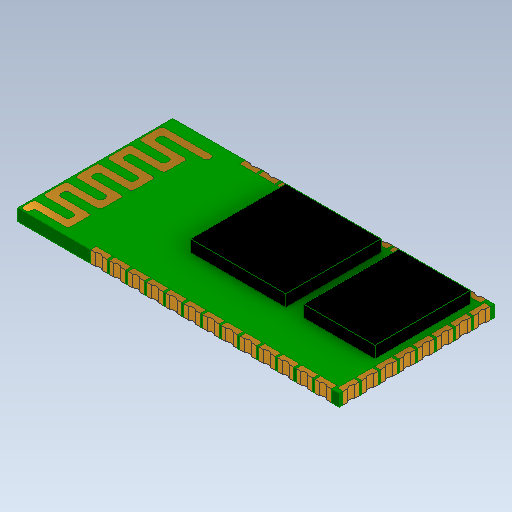
# Autodesk Inventor part: HC-05
Saved by Autodesk Inventor 2020 (Build 240168000, 168)
## iProperties
Created: 2019-12-28
Part Number: HC-05
Material: Generic
Document SubType Name: Modeling
Designer: ermoz
Density: 1 g/cm^3
Appearance: Default
Mass: 0.461242 g
Surface Area: 10.6929 cm^2
Volume: 0.461242 cm^3
Author: ermoz
Autodesk Inventor part; units mm, degrees
ref_plane "YZ Plane" through (0, 0, 0) normal (1, 0, 0) x (0, 1, 0)
ref_plane "XZ Plane" through (0, 0, 0) normal (0, 1, 0) x (-1, 0, 0)
ref_plane "XY Plane" through (0, 0, 0) normal (0, 0, 1) x (1, 0, 0)
sketch "Sketch1" plane through (0, 0, 0) normal (0, 1, 0) x (-1, 0, 0)
  line L0 (0, 0) -> (-27, 0)
  line L1 (-27, 0) -> (-27, -13)
  line L2 (-27, -13) -> (0, -13)
  line L3 (0, -13) -> (0, 0)
  dimension "d0" = 27
  dimension "d1" = 13
  constraints: 8 end point, 2 parallel, 1 horizontal, 1 perpendicular
  measures "d0" distance of L2.end L1.end
  measures "d1" distance of L1.end L0.end
extrude "Extrusion1" add sketch "Sketch1" along normal blind 1
sketch "Sketch2" plane through (0, 1, 0) normal (0, 1, 0) x (1, 0, 0)
  line L0 (27, 6.215) -> (26.5, 6.785) construction
  line L1 (26.5, 6.215) -> (27, 6.785) construction
  line L2 (26.5, 6.785) -> (26.5, 7.785)
  line L3 (26.5, 8.355) -> (26.5, 9.355)
  line L4 (26.5, 9.925) -> (26.5, 10.925)
  line L5 (26.5, 11.495) -> (26.5, 12.495)
  line L6 (27, 6.785) -> (27, 6.985)
  line L7 (27, 7.785) -> (27, 7.585)
  arc A0 (27, 7.585) -> (27, 6.985) centre (27.2975, 7.285) ccw
  line L8 (27, 8.355) -> (27, 8.555)
  line L9 (27, 9.355) -> (27, 9.155)
  arc A1 (27, 9.155) -> (27, 8.555) centre (27.2975, 8.855) ccw
  line L10 (27, 9.925) -> (27, 10.125)
  line L11 (27, 10.925) -> (27, 10.725)
  arc A2 (27, 10.725) -> (27, 10.125) centre (27.2975, 10.425) ccw
  line L12 (27, 11.495) -> (27, 11.695)
  line L13 (27, 12.495) -> (27, 12.295)
  arc A3 (27, 12.295) -> (27, 11.695) centre (27.2975, 11.995) ccw
  line L14 (26.5, 6.215) -> (26.5, 5.215)
  line L15 (26.5, 4.645) -> (26.5, 3.645)
  line L16 (26.5, 3.075) -> (26.5, 2.075)
  line L17 (26.5, 1.505) -> (26.5, 0.505)
  arc A4 (27, 6.015) -> (27, 5.415) centre (27.2975, 5.715) ccw
  arc A5 (27, 4.445) -> (27, 3.845) centre (27.2975, 4.145) ccw
  arc A6 (27, 2.875) -> (27, 2.275) centre (27.2975, 2.575) ccw
  arc A7 (27, 1.305) -> (27, 0.705) centre (27.2975, 1.005) ccw
  line L18 (27, 0.505) -> (27, 0.705)
  line L19 (27, 1.305) -> (27, 1.505)
  line L20 (27, 2.075) -> (27, 2.275)
  line L21 (27, 2.875) -> (27, 3.075)
  line L22 (27, 3.645) -> (27, 3.845)
  line L23 (27, 4.445) -> (27, 4.645)
  line L24 (27, 5.215) -> (27, 5.415)
  line L25 (27, 6.015) -> (27, 6.215)
  line L26 (27, 6.785) -> (27, 6.985)
  line L27 (27, 7.585) -> (27, 7.785)
  line L28 (27, 8.355) -> (27, 8.555)
  line L29 (27, 9.155) -> (27, 9.355)
  line L30 (27, 9.925) -> (27, 10.125)
  line L31 (27, 10.725) -> (27, 10.925)
  line L32 (27, 11.495) -> (27, 11.695)
  line L33 (27, 12.295) -> (27, 12.495)
  line L34 (27, 0.305) -> (26.5, 0.305)
  line L35 (26.5, 0.305) -> (26.5, 1.705)
  line L36 (26.5, 1.705) -> (27, 1.705)
  line L37 (27, 0.305) -> (26.5, 1.705) construction
  line L38 (26.5, 0.305) -> (27, 1.705) construction
  line L39 (27, 1.875) -> (26.5, 1.875)
  line L40 (26.5, 1.875) -> (26.5, 3.275)
  line L41 (26.5, 3.275) -> (27, 3.275)
  line L42 (27, 1.875) -> (26.5, 3.275) construction
  line L43 (26.5, 1.875) -> (27, 3.275) construction
  line L44 (27, 3.445) -> (26.5, 3.445)
  line L45 (26.5, 3.445) -> (26.5, 4.845)
  line L46 (26.5, 4.845) -> (27, 4.845)
  line L47 (27, 3.445) -> (26.5, 4.845) construction
  line L48 (26.5, 3.445) -> (27, 4.845) construction
  line L49 (27, 5.015) -> (26.5, 5.015)
  line L50 (26.5, 5.015) -> (26.5, 6.415)
  line L51 (26.5, 6.415) -> (27, 6.415)
  line L52 (27, 5.015) -> (26.5, 6.415) construction
  line L53 (26.5, 5.015) -> (27, 6.415) construction
  line L54 (27, 6.585) -> (26.5, 6.585)
  line L55 (26.5, 6.585) -> (26.5, 7.985)
  line L56 (26.5, 7.985) -> (27, 7.985)
  line L57 (27, 6.585) -> (26.5, 7.985) construction
  line L58 (26.5, 6.585) -> (27, 7.985) construction
  line L59 (27, 8.155) -> (26.5, 8.155)
  line L60 (26.5, 8.155) -> (26.5, 9.555)
  line L61 (26.5, 9.555) -> (27, 9.555)
  line L62 (27, 8.155) -> (26.5, 9.555) construction
  line L63 (26.5, 8.155) -> (27, 9.555) construction
  line L64 (27, 9.725) -> (26.5, 9.725)
  line L65 (26.5, 9.725) -> (26.5, 11.125)
  line L66 (26.5, 11.125) -> (27, 11.125)
  line L67 (27, 9.725) -> (26.5, 11.125) construction
  line L68 (26.5, 9.725) -> (27, 11.125) construction
  line L69 (27, 11.295) -> (26.5, 11.295)
  line L70 (26.5, 11.295) -> (26.5, 12.695)
  line L71 (26.5, 12.695) -> (27, 12.695)
  line L72 (27, 11.295) -> (26.5, 12.695) construction
  line L73 (26.5, 11.295) -> (27, 12.695) construction
  line L74 (27, 1.705) -> (27, 1.305)
  line L75 (27, 0.705) -> (27, 0.305)
  line L76 (27, 1.875) -> (27, 2.275)
  line L77 (27, 2.875) -> (27, 3.275)
  line L78 (27, 3.445) -> (27, 3.845)
  line L79 (27, 4.445) -> (27, 4.845)
  line L80 (27, 5.015) -> (27, 5.415)
  line L81 (27, 6.015) -> (27, 6.415)
  line L82 (27, 6.585) -> (27, 6.985)
  line L83 (27, 7.585) -> (27, 7.985)
  line L84 (27, 8.155) -> (27, 8.555)
  line L85 (27, 9.155) -> (27, 9.555)
  line L86 (27, 9.725) -> (27, 10.125)
  line L87 (27, 10.725) -> (27, 11.125)
  line L88 (27, 11.295) -> (27, 11.695)
  line L89 (27, 12.295) -> (27, 12.695)
  arc A8 (27, 1.305) -> (27, 0.705) centre (27.2975, 1.005) ccw
  arc A9 (27, 2.875) -> (27, 2.275) centre (27.2975, 2.575) ccw
  arc A10 (27, 4.445) -> (27, 3.845) centre (27.2975, 4.145) ccw
  arc A11 (27, 6.015) -> (27, 5.415) centre (27.2975, 5.715) ccw
  arc A12 (27, 7.585) -> (27, 6.985) centre (27.2975, 7.285) ccw
  arc A13 (27, 9.155) -> (27, 8.555) centre (27.2975, 8.855) ccw
  arc A14 (27, 10.725) -> (27, 10.125) centre (27.2975, 10.425) ccw
  line L90 (27, 0) -> (27, 13) projected
  arc A15 (27, 12.295) -> (27, 11.695) centre (27.2975, 11.995) ccw
  line L91 (27, 0.305) -> (27, 12.695)
  point P0 (0, 0)
  point P1 (26.75, 1.005)
  point P2 (26.75, 2.575)
  point P3 (26.75, 4.145)
  point P4 (26.75, 5.715)
  point P5 (26.75, 7.285)
  point P6 (26.75, 8.855)
  point P7 (26.75, 10.425)
  point P8 (26.75, 11.995)
  dimension "d6" = 0.57
  dimension "d8" = 1
  dimension "d12" = 1
  dimension "d16" = 1
  dimension "d19" = 0.5
  dimension "d20" = 1
  dimension "d22" = 0.2
  dimension "d23" = 0.2
  dimension "d24" = 0.2
  dimension "d25" = 0.2
  dimension "d29" = 1.4
  dimension "d30" = 1.4
  dimension "d31" = 1.4
  dimension "d32" = 1.4
  dimension "d33" = 1.4
  dimension "d34" = 1.4
  dimension "d35" = 1.4
  dimension "d36" = 1.4
  constraints: 182 end point, 32 point on circle, 16 centre point, 16 midpoint, 15 collinear, 8 coincident, 8 horizontal, 8 parallel, 8 perpendicular, 3 point on line, 1 vertical, 2 other
  measures "d6" distance of L1.start L0.end
  measures "d8" distance of L2.start L2.end
  measures "d12" distance of L3.start L3.end
  measures "d16" distance of L4.start L4.end
  measures "d19" distance of L5.end L13.start
  measures "d20" distance of L5.start L5.end
  measures "d22" distance of L7.start L7.end
  measures "d23" distance of L8.start L8.end
  measures "d24" distance of L9.start L9.end
  measures "d25" distance of L10.start L10.end
  measures "d29" distance of L34.end L35.end
  measures "d30" distance of L39.end L40.end
  measures "d31" distance of L44.end L45.end
  measures "d32" distance of L49.end L50.end
  measures "d33" distance of L54.end L55.end
  measures "d34" distance of L59.end L60.end
  measures "d35" distance of L64.end L65.end
  measures "d36" distance of L69.end L70.end
extrude "Extrusion2" cut sketch "Sketch2" against normal blind 1 contours L69 L70 L5 L71 L89 L13 A3 L12 L88 | L64 L65 L4 L66 L87 L11 A2 L10 L86 | L59 L60 L3 L61 L85 L9 A1 L8 L84 | L74 L19 A7 L18 L75 L34 L35 L17 L36 | L77 L21 A6 L20 L76 L39 L40 L16 L41 | L79 L23 A5 L22 L78 L44 L45 L15 L46 | L81 L25 A4 L24 L80 L49 L50 L14 L51 | L2 L55 L56 L83 L7 A0 L6 L82 L54
extrude "Extrusion3" add sketch "Sketch2" against normal blind 1 separate body contours L69 L70 L5 L71 L89 L13 A3 L12 L88 | L64 L65 L4 L66 L87 L11 A2 L10 L86 | L59 L60 L3 L61 L85 L9 A1 L8 L84 | L74 L19 A7 L18 L75 L34 L35 L17 L36 | L77 L21 A6 L20 L76 L39 L40 L16 L41 | L79 L23 A5 L22 L78 L44 L45 L15 L46 | L81 L25 A4 L24 L80 L49 L50 L14 L51 | L2 L55 L56 L83 L7 A0 L6 L82 L54
sketch "Sketch3" plane through (0, 1, 0) normal (0, 1, 0) x (1, 0, 0)
  line L0 (26.7293, 0.5191) -> (27.1446, 0.5191)
  line L1 (27.1446, 0.5191) -> (27.1446, 1.5386)
  line L2 (27.1446, 1.5386) -> (26.7293, 1.5386)
  line L3 (26.7293, 1.5386) -> (26.7293, 0.5191)
  line L4 (26.7293, 2.1711) -> (27.1446, 2.1711)
  line L5 (27.1446, 2.1711) -> (27.1446, 3.0584)
  line L6 (27.1446, 3.0584) -> (26.7293, 3.0584)
  line L7 (26.7293, 3.0584) -> (26.7293, 2.1711)
  line L8 (26.7293, 3.7192) -> (27.088, 3.7192)
  line L9 (27.088, 3.7192) -> (27.088, 4.616)
  line L10 (27.088, 4.616) -> (26.7293, 4.616)
  line L11 (26.7293, 4.616) -> (26.7293, 3.7192)
  line L12 (26.7293, 5.305) -> (27.1446, 5.305)
  line L13 (27.1446, 5.305) -> (27.1446, 6.1546)
  line L14 (27.1446, 6.1546) -> (26.7293, 6.1546)
  line L15 (26.7293, 6.1546) -> (26.7293, 5.305)
  line L16 (26.7293, 6.9192) -> (27.1446, 6.9192)
  line L17 (27.1446, 6.9192) -> (27.1446, 7.7122)
  line L18 (27.1446, 7.7122) -> (26.7293, 7.7122)
  line L19 (26.7293, 7.7122) -> (26.7293, 6.9192)
  line L20 (26.7293, 8.4673) -> (27.239, 8.4673)
  line L21 (27.239, 8.4673) -> (27.239, 9.3358)
  line L22 (27.239, 9.3358) -> (26.7293, 9.3358)
  line L23 (26.7293, 9.3358) -> (26.7293, 8.4673)
  line L24 (26.6726, 9.9966) -> (27.239, 9.9966)
  line L25 (27.239, 9.9966) -> (27.239, 10.8556)
  line L26 (27.239, 10.8556) -> (26.6726, 10.8556)
  line L27 (26.6726, 10.8556) -> (26.6726, 9.9966)
  line L28 (26.6726, 11.5541) -> (27.239, 11.5541)
  line L29 (27.239, 11.5541) -> (27.239, 12.517)
  line L30 (27.239, 12.517) -> (26.6726, 12.517)
  line L31 (26.6726, 12.517) -> (26.6726, 11.5541)
  point P0 (0, 0)
  constraints: 64 end point, 16 parallel, 11 point on line, 8 horizontal, 8 perpendicular
extrude "Extrusion4" cut sketch "Sketch3" against normal blind 1 bodies 1
sketch "Sketch4" plane through (0, 1, 0) normal (0, 1, 0) x (1, 0, 0)
  line L0 (24.93, 13) -> (24.93, 12.5)
  line L1 (24.93, 12.5) -> (26.33, 12.5)
  line L2 (26.33, 12.5) -> (26.33, 13)
  line L3 (23.36, 13) -> (23.36, 12.5)
  line L4 (23.36, 12.5) -> (24.76, 12.5)
  line L5 (24.76, 12.5) -> (24.76, 13)
  line L6 (21.79, 13) -> (21.79, 12.5)
  line L7 (21.79, 12.5) -> (23.19, 12.5)
  line L8 (23.19, 12.5) -> (23.19, 13)
  line L9 (20.22, 13) -> (20.22, 12.5)
  line L10 (20.22, 12.5) -> (21.62, 12.5)
  line L11 (21.62, 12.5) -> (21.62, 13)
  line L12 (18.65, 13) -> (18.65, 12.5)
  line L13 (18.65, 12.5) -> (20.05, 12.5)
  line L14 (20.05, 12.5) -> (20.05, 13)
  line L15 (17.08, 13) -> (17.08, 12.5)
  line L16 (17.08, 12.5) -> (18.48, 12.5)
  line L17 (18.48, 12.5) -> (18.48, 13)
  line L18 (15.51, 13) -> (15.51, 12.5)
  line L19 (15.51, 12.5) -> (16.91, 12.5)
  line L20 (16.91, 12.5) -> (16.91, 13)
  line L21 (13.94, 13) -> (13.94, 12.5)
  line L22 (13.94, 12.5) -> (15.34, 12.5)
  line L23 (15.34, 12.5) -> (15.34, 13)
  line L24 (12.37, 13) -> (12.37, 12.5)
  line L25 (12.37, 12.5) -> (13.77, 12.5)
  line L26 (13.77, 12.5) -> (13.77, 13)
  line L27 (10.8, 13) -> (10.8, 12.5)
  line L28 (10.8, 12.5) -> (12.2, 12.5)
  line L29 (12.2, 12.5) -> (12.2, 13)
  line L30 (9.23, 13) -> (9.23, 12.5)
  line L31 (9.23, 12.5) -> (10.63, 12.5)
  line L32 (10.63, 12.5) -> (10.63, 13)
  line L33 (7.66, 13) -> (7.66, 12.5)
  line L34 (7.66, 12.5) -> (9.06, 12.5)
  line L35 (9.06, 12.5) -> (9.06, 13)
  line L36 (6.09, 13) -> (6.09, 12.5)
  line L37 (6.09, 12.5) -> (7.49, 12.5)
  line L38 (7.49, 12.5) -> (7.49, 13)
  line L39 (26.33, 13) -> (25.93, 13)
  line L40 (24.93, 13) -> (25.33, 13)
  line L41 (24.76, 13) -> (24.36, 13)
  line L42 (23.36, 13) -> (23.76, 13)
  line L43 (23.19, 13) -> (22.79, 13)
  line L44 (21.79, 13) -> (22.19, 13)
  line L45 (21.62, 13) -> (21.22, 13)
  line L46 (20.22, 13) -> (20.62, 13)
  line L47 (20.05, 13) -> (19.65, 13)
  line L48 (18.65, 13) -> (19.05, 13)
  line L49 (18.48, 13) -> (18.08, 13)
  line L50 (17.08, 13) -> (17.48, 13)
  line L51 (16.91, 13) -> (16.51, 13)
  line L52 (15.51, 13) -> (15.91, 13)
  line L53 (15.34, 13) -> (14.94, 13)
  line L54 (13.94, 13) -> (14.34, 13)
  line L55 (13.77, 13) -> (13.37, 13)
  line L56 (12.37, 13) -> (12.77, 13)
  line L57 (12.2, 13) -> (11.8, 13)
  line L58 (10.8, 13) -> (11.2, 13)
  line L59 (10.63, 13) -> (10.23, 13)
  line L60 (9.23, 13) -> (9.63, 13)
  line L61 (9.06, 13) -> (8.66, 13)
  line L62 (7.66, 13) -> (8.06, 13)
  line L63 (7.49, 13) -> (7.09, 13)
  line L64 (6.09, 13) -> (6.49, 13)
  line L65 (6.09, 13) -> (6.09, 12.875)
  arc A0 (25.33, 13) -> (25.93, 13) centre (25.63, 13.2975) ccw
  arc A1 (23.76, 13) -> (24.36, 13) centre (24.06, 13.2975) ccw
  arc A2 (22.19, 13) -> (22.79, 13) centre (22.49, 13.2975) ccw
  arc A3 (20.62, 13) -> (21.22, 13) centre (20.92, 13.2975) ccw
  arc A4 (19.05, 13) -> (19.65, 13) centre (19.35, 13.2975) ccw
  arc A5 (17.48, 13) -> (18.08, 13) centre (17.78, 13.2975) ccw
  arc A6 (15.91, 13) -> (16.51, 13) centre (16.21, 13.2975) ccw
  arc A7 (14.34, 13) -> (14.94, 13) centre (14.64, 13.2975) ccw
  arc A8 (12.77, 13) -> (13.37, 13) centre (13.07, 13.2975) ccw
  arc A9 (11.2, 13) -> (11.8, 13) centre (11.5, 13.2975) ccw
  arc A10 (9.63, 13) -> (10.23, 13) centre (9.93, 13.2975) ccw
  arc A11 (8.06, 13) -> (8.66, 13) centre (8.36, 13.2975) ccw
  arc A12 (6.49, 13) -> (7.09, 13) centre (6.79, 13.2975) ccw
  line L66 (0, 13) -> (0, 0) projected
  line L67 (0, 6.5) -> (5.1876, 6.5)
  line L68 (24.93, 0) -> (24.93, 0.5)
  line L69 (24.93, 0.5) -> (26.33, 0.5)
  line L70 (26.33, 0.5) -> (26.33, 0)
  line L71 (23.36, 0) -> (23.36, 0.5)
  line L72 (23.36, 0.5) -> (24.76, 0.5)
  line L73 (24.76, 0.5) -> (24.76, 0)
  line L74 (21.79, 0) -> (21.79, 0.5)
  line L75 (21.79, 0.5) -> (23.19, 0.5)
  line L76 (23.19, 0.5) -> (23.19, 0)
  line L77 (20.22, 0) -> (20.22, 0.5)
  line L78 (20.22, 0.5) -> (21.62, 0.5)
  line L79 (21.62, 0.5) -> (21.62, 0)
  line L80 (18.65, 0) -> (18.65, 0.5)
  line L81 (18.65, 0.5) -> (20.05, 0.5)
  line L82 (20.05, 0.5) -> (20.05, 0)
  line L83 (17.08, 0) -> (17.08, 0.5)
  line L84 (17.08, 0.5) -> (18.48, 0.5)
  line L85 (18.48, 0.5) -> (18.48, 0)
  line L86 (15.51, 0) -> (15.51, 0.5)
  line L87 (15.51, 0.5) -> (16.91, 0.5)
  line L88 (16.91, 0.5) -> (16.91, 0)
  line L89 (13.94, 0) -> (13.94, 0.5)
  line L90 (13.94, 0.5) -> (15.34, 0.5)
  line L91 (15.34, 0.5) -> (15.34, 0)
  line L92 (12.37, 0) -> (12.37, 0.5)
  line L93 (12.37, 0.5) -> (13.77, 0.5)
  line L94 (13.77, 0.5) -> (13.77, 0)
  line L95 (10.8, 0.5) -> (12.2, 0.5)
  line L96 (12.2, 0.5) -> (12.2, 0)
  line L97 (9.23, 0) -> (9.23, 0.5)
  line L98 (9.23, 0.5) -> (10.63, 0.5)
  line L99 (10.63, 0.5) -> (10.63, 0)
  line L100 (7.66, 0) -> (7.66, 0.5)
  line L101 (7.66, 0.5) -> (9.06, 0.5)
  line L102 (9.06, 0.5) -> (9.06, 0)
  line L103 (6.09, 0) -> (6.09, 0.5)
  line L104 (6.09, 0.5) -> (7.49, 0.5)
  line L105 (7.49, 0.5) -> (7.49, 0)
  line L106 (26.33, 0) -> (25.93, 0)
  line L107 (24.93, 0) -> (25.33, 0)
  line L108 (24.76, 0) -> (24.36, 0)
  line L109 (23.36, 0) -> (23.76, 0)
  line L110 (23.19, 0) -> (22.79, 0)
  line L111 (21.79, 0) -> (22.19, 0)
  line L112 (21.62, 0) -> (21.22, 0)
  line L113 (20.22, 0) -> (20.62, 0)
  line L114 (20.05, 0) -> (19.65, 0)
  line L115 (18.65, 0) -> (19.05, 0)
  line L116 (18.48, 0) -> (18.08, 0)
  line L117 (17.08, 0) -> (17.48, 0)
  line L118 (16.91, 0) -> (16.51, 0)
  line L119 (15.51, 0) -> (15.91, 0)
  line L120 (15.34, 0) -> (14.94, 0)
  line L121 (13.94, 0) -> (14.34, 0)
  line L122 (13.77, 0) -> (13.37, 0)
  line L123 (12.37, 0) -> (12.77, 0)
  line L124 (12.2, 0) -> (11.8, 0)
  line L125 (10.8, 0) -> (11.2, 0)
  line L126 (10.63, 0) -> (10.23, 0)
  line L127 (9.23, 0) -> (9.63, 0)
  line L128 (9.06, 0) -> (8.66, 0)
  line L129 (7.66, 0) -> (8.06, 0)
  line L130 (7.49, 0) -> (7.09, 0)
  line L131 (6.09, 0) -> (6.49, 0)
  arc A13 (25.93, 0) -> (25.33, 0) centre (25.63, -0.2975) ccw
  arc A14 (24.36, 0) -> (23.76, 0) centre (24.06, -0.2975) ccw
  arc A15 (22.79, 0) -> (22.19, 0) centre (22.49, -0.2975) ccw
  arc A16 (21.22, 0) -> (20.62, 0) centre (20.92, -0.2975) ccw
  arc A17 (19.65, 0) -> (19.05, 0) centre (19.35, -0.2975) ccw
  arc A18 (18.08, 0) -> (17.48, 0) centre (17.78, -0.2975) ccw
  arc A19 (16.51, 0) -> (15.91, 0) centre (16.21, -0.2975) ccw
  arc A20 (14.94, 0) -> (14.34, 0) centre (14.64, -0.2975) ccw
  arc A21 (13.37, 0) -> (12.77, 0) centre (13.07, -0.2975) ccw
  arc A22 (11.8, 0) -> (11.2, 0) centre (11.5, -0.2975) ccw
  arc A23 (10.23, 0) -> (9.63, 0) centre (9.93, -0.2975) ccw
  arc A24 (8.66, 0) -> (8.06, 0) centre (8.36, -0.2975) ccw
  arc A25 (7.09, 0) -> (6.49, 0) centre (6.79, -0.2975) ccw
  line L132 (10.8, 0) -> (10.8, 0.5)
  line L133 (0, 0) -> (27, 0) projected
  dimension "d46" = 0.17
  dimension "d47" = 1.4
  dimension "d49" = 0.17
  dimension "d50" = 1.4
  dimension "d52" = 0.17
  dimension "d53" = 1.4
  dimension "d55" = 0.17
  dimension "d56" = 1.4
  dimension "d58" = 0.17
  dimension "d59" = 1.4
  dimension "d61" = 0.17
  dimension "d62" = 1.4
  dimension "d64" = 0.17
  dimension "d65" = 1.4
  dimension "d67" = 0.17
  dimension "d68" = 1.4
  dimension "d70" = 0.17
  dimension "d71" = 1.4
  dimension "d73" = 0.17
  dimension "d74" = 1.4
  dimension "d76" = 0.17
  dimension "d77" = 1.4
  dimension "d80" = 1.4
  dimension "d81" = 0.5
  dimension "d82" = 0.4
  dimension "d83" = 0.4
  dimension "d84" = 0.4
  dimension "d85" = 0.4
  dimension "d86" = 0.4
  dimension "d87" = 0.4
  dimension "d88" = 0.4
  dimension "d89" = 0.4
  dimension "d90" = 0.4
  dimension "d91" = 0.4
  dimension "d92" = 0.4
  dimension "d93" = 0.4
  dimension "d94" = 0.4
  dimension "d95" = 0.4
  dimension "d96" = 0.4
  dimension "d97" = 0.4
  dimension "d98" = 0.4
  dimension "d99" = 0.4
  dimension "d100" = 0.4
  dimension "d101" = 0.4
  dimension "d102" = 0.4
  dimension "d103" = 0.4
  dimension "d104" = 0.4
  dimension "d105" = 0.4
  dimension "d106" = 0.4
  dimension "d107" = 0.4
  dimension "d108" = 0.125
  constraints: 264 end point, 91 symmetric about line, 52 point on circle, 26 centre point, 13 parallel, 1 horizontal, 1 midpoint, 1 point on line, 1 vertical, 14 other
  measures "d46" distance of L0.start L5.end
  measures "d47" distance of L4.end L3.end
  measures "d49" distance of L3.start L8.end
  measures "d50" distance of L7.end L6.end
  measures "d52" distance of L6.start L11.end
  measures "d53" distance of L10.end L9.end
  measures "d55" distance of L9.start L14.end
  measures "d56" distance of L13.end L12.end
  measures "d58" distance of L12.start L17.end
  measures "d59" distance of L16.end L15.end
  measures "d61" distance of L15.start L20.end
  measures "d62" distance of L19.end L18.end
  measures "d64" distance of L18.start L23.end
  measures "d65" distance of L22.end L21.end
  measures "d67" distance of L21.start L26.end
  measures "d68" distance of L25.end L24.end
  measures "d70" distance of L24.start L29.end
  measures "d71" distance of L28.end L27.end
  measures "d73" distance of L27.start L32.end
  measures "d74" distance of L31.end L30.end
  measures "d76" distance of L30.start L35.end
  measures "d77" distance of L34.end L33.end
  measures "d80" distance of L37.end L36.end
  measures "d81" distance of L36.end L36.start
  measures "d82" distance of L2.end L39.end
  measures "d83" distance of L0.start L40.end
  measures "d84" distance of L5.end L41.end
  measures "d85" distance of L3.start L42.end
  measures "d86" distance of L8.end L43.end
  measures "d87" distance of L6.start L44.end
  measures "d88" distance of L11.end L45.end
  measures "d89" distance of L9.start L46.end
  measures "d90" distance of L14.end L47.end
  measures "d91" distance of L12.start L48.end
  measures "d92" distance of L17.end L49.end
  measures "d93" distance of L15.start L50.end
  measures "d94" distance of L20.end L51.end
  measures "d95" distance of L18.start L52.end
  measures "d96" distance of L23.end L53.end
  measures "d97" distance of L21.start L54.end
  measures "d98" distance of L26.end L55.end
  measures "d99" distance of L24.start L56.end
  measures "d100" distance of L29.end L57.end
  measures "d101" distance of L27.start L58.end
  measures "d102" distance of L32.end L59.end
  measures "d103" distance of L30.start L60.end
  measures "d104" distance of L35.end L61.end
  measures "d105" distance of L33.start L62.end
  measures "d106" distance of L38.end L63.end
  measures "d107" distance of L36.start L64.end
  measures "d108" distance of L36.start L65.end
extrude "Extrusion5" cut sketch "Sketch4" against normal blind 1 contours L40 A0 L39 L2 L1 L0 | L42 A1 L41 L5 L4 L3 | L44 A2 L43 L8 L7 L6 | L46 A3 L45 L11 L10 L9 | L48 A4 L47 L14 L13 L12 | L50 A5 L49 L17 L16 L15 | L52 A6 L51 L20 L19 L18 | L54 A7 L53 L23 L22 L21 | L56 A8 L55 L26 L25 L24 | L58 A9 L57 L29 L28 L27 | L60 A10 L59 L32 L31 L30 | L62 A11 L61 L35 L34 L33 | L64 A12 L63 L38 L37 L36 | L68 L69 L70 L106 A13 L107 | L130 A25 L131 L103 L104 L105 | L128 A24 L129 L100 L101 L102 | L126 A23 L127 L97 L98 L99 | L124 A22 L125 L132 L95 L96 | L122 A21 L123 L92 L93 L94 | L120 A20 L121 L89 L90 L91 | L118 A19 L119 L86 L87 L88 | L116 A18 L117 L83 L84 L85 | L114 A17 L115 L80 L81 L82 | L112 A16 L113 L77 L78 L79 | L110 A15 L111 L74 L75 L76 | L108 A14 L109 L71 L72 L73 bodies 1
extrude "Extrusion6" add sketch "Sketch4" against normal blind 1 separate body contours L40 A0 L39 L2 L1 L0 | L42 A1 L41 L5 L4 L3 | L44 A2 L43 L8 L7 L6 | L46 A3 L45 L11 L10 L9 | L48 A4 L47 L14 L13 L12 | L50 A5 L49 L17 L16 L15 | L52 A6 L51 L20 L19 L18 | L54 A7 L53 L23 L22 L21 | L56 A8 L55 L26 L25 L24 | L58 A9 L57 L29 L28 L27 | L60 A10 L59 L32 L31 L30 | L62 A11 L61 L35 L34 L33 | L64 A12 L63 L38 L37 L36 | L68 L69 L70 L106 A13 L107 | L130 A25 L131 L103 L104 L105 | L128 A24 L129 L100 L101 L102 | L126 A23 L127 L97 L98 L99 | L124 A22 L125 L132 L95 L96 | L122 A21 L123 L92 L93 L94 | L120 A20 L121 L89 L90 L91 | L118 A19 L119 L86 L87 L88 | L116 A18 L117 L83 L84 L85 | L114 A17 L115 L80 L81 L82 | L112 A16 L113 L77 L78 L79 | L110 A15 L111 L74 L75 L76 | L108 A14 L109 L71 L72 L73
sketch "Sketch5" plane through (0, 1, 0) normal (0, 1, 0) x (1, 0, 0)
  line L0 (6.3703, 13.1269) -> (7.3266, 13.1269)
  line L1 (7.3266, 13.1269) -> (7.3266, 12.766)
  line L2 (7.3266, 12.766) -> (6.3703, 12.766)
  line L3 (6.3703, 12.766) -> (6.3703, 13.1269)
  line L4 (7.904, 13.1269) -> (8.9866, 13.1269)
  line L5 (8.9866, 13.1269) -> (8.9866, 12.766)
  line L6 (8.9866, 12.766) -> (7.904, 12.766)
  line L7 (7.904, 12.766) -> (7.904, 13.1269)
  line L8 (9.4918, 13.2352) -> (10.5564, 13.2352)
  line L9 (10.5564, 13.2352) -> (10.5564, 12.766)
  line L10 (10.5564, 12.766) -> (9.4918, 12.766)
  line L11 (9.4918, 12.766) -> (9.4918, 13.2352)
  line L12 (11.0616, 13.2352) -> (11.9638, 13.2352)
  line L13 (11.9638, 13.2352) -> (11.9638, 12.766)
  line L14 (11.9638, 12.766) -> (11.0616, 12.766)
  line L15 (11.0616, 12.766) -> (11.0616, 13.2352)
  line L16 (12.5592, 13.2352) -> (13.6419, 13.2352)
  line L17 (13.6419, 13.2352) -> (13.6419, 12.6217)
  line L18 (13.6419, 12.6217) -> (12.5592, 12.6217)
  line L19 (12.5592, 12.6217) -> (12.5592, 13.2352)
  line L20 (14.2553, 13.2352) -> (15.1214, 13.2352)
  line L21 (15.1214, 13.2352) -> (15.1214, 12.766)
  line L22 (15.1214, 12.766) -> (14.2553, 12.766)
  line L23 (14.2553, 12.766) -> (14.2553, 13.2352)
  line L24 (15.7891, 13.2352) -> (16.6732, 13.2352)
  line L25 (16.6732, 13.2352) -> (16.6732, 12.766)
  line L26 (16.6732, 12.766) -> (15.7891, 12.766)
  line L27 (15.7891, 12.766) -> (15.7891, 13.2352)
  line L28 (17.3769, 13.2352) -> (18.225, 13.2352)
  line L29 (18.225, 13.2352) -> (18.225, 12.766)
  line L30 (18.225, 12.766) -> (17.3769, 12.766)
  line L31 (17.3769, 12.766) -> (17.3769, 13.2352)
  line L32 (18.8204, 13.2352) -> (19.903, 13.2352)
  line L33 (19.903, 13.2352) -> (19.903, 12.766)
  line L34 (19.903, 12.766) -> (18.8204, 12.766)
  line L35 (18.8204, 12.766) -> (18.8204, 13.2352)
  line L36 (20.4263, 13.2352) -> (21.5269, 13.2352)
  line L37 (21.5269, 13.2352) -> (21.5269, 12.766)
  line L38 (21.5269, 12.766) -> (20.4263, 12.766)
  line L39 (20.4263, 12.766) -> (20.4263, 13.2352)
  line L40 (22.0322, 13.2352) -> (23.0065, 13.2352)
  line L41 (23.0065, 13.2352) -> (23.0065, 12.766)
  line L42 (23.0065, 12.766) -> (22.0322, 12.766)
  line L43 (22.0322, 12.766) -> (22.0322, 13.2352)
  line L44 (23.6381, 13.2352) -> (24.5222, 13.2352)
  line L45 (24.5222, 13.2352) -> (24.5222, 12.766)
  line L46 (24.5222, 12.766) -> (23.6381, 12.766)
  line L47 (23.6381, 12.766) -> (23.6381, 13.2352)
  line L48 (25.13, 13.2352) -> (26.1281, 13.2352)
  line L49 (26.1281, 13.2352) -> (26.1281, 12.766)
  line L50 (26.1281, 12.766) -> (25.13, 12.766)
  line L51 (25.13, 12.766) -> (25.13, 13.2352)
  line L52 (6.2439, -0.2615) -> (7.3266, -0.2615)
  line L53 (7.3266, -0.2615) -> (7.3266, 0.2618)
  line L54 (7.3266, 0.2618) -> (6.2439, 0.2618)
  line L55 (6.2439, 0.2618) -> (6.2439, -0.2615)
  line L56 (7.904, 0.2618) -> (8.8964, 0.2618)
  line L57 (8.8964, 0.2618) -> (8.8964, -0.3878)
  line L58 (8.8964, -0.3878) -> (7.904, -0.3878)
  line L59 (7.904, -0.3878) -> (7.904, 0.2618)
  line L60 (9.4918, 0.2618) -> (10.4301, 0.2618)
  line L61 (10.4301, 0.2618) -> (10.4301, -0.3878)
  line L62 (10.4301, -0.3878) -> (9.4918, -0.3878)
  line L63 (9.4918, -0.3878) -> (9.4918, 0.2618)
  line L64 (11.0616, 0.2618) -> (12.0901, 0.2618)
  line L65 (12.0901, 0.2618) -> (12.0901, -0.2615)
  line L66 (12.0901, -0.2615) -> (11.0616, -0.2615)
  line L67 (11.0616, -0.2615) -> (11.0616, 0.2618)
  line L68 (12.5592, 0.2618) -> (13.6419, 0.2618)
  line L69 (13.6419, 0.2618) -> (13.6419, -0.2615)
  line L70 (13.6419, -0.2615) -> (12.5592, -0.2615)
  line L71 (12.5592, -0.2615) -> (12.5592, 0.2618)
  line L72 (14.2553, 0.2618) -> (15.1214, 0.2618)
  line L73 (15.1214, 0.2618) -> (15.1214, -0.2615)
  line L74 (15.1214, -0.2615) -> (14.2553, -0.2615)
  line L75 (14.2553, -0.2615) -> (14.2553, 0.2618)
  line L76 (15.7891, 0.2618) -> (16.6732, 0.2618)
  line L77 (16.6732, 0.2618) -> (16.6732, -0.3878)
  line L78 (16.6732, -0.3878) -> (15.7891, -0.3878)
  line L79 (15.7891, -0.3878) -> (15.7891, 0.2618)
  line L80 (17.3769, 0.2618) -> (18.3332, 0.2618)
  line L81 (18.3332, 0.2618) -> (18.3332, -0.3878)
  line L82 (18.3332, -0.3878) -> (17.3769, -0.3878)
  line L83 (17.3769, -0.3878) -> (17.3769, 0.2618)
  line L84 (18.8204, 0.2618) -> (19.903, 0.2618)
  line L85 (19.903, 0.2618) -> (19.903, -0.3878)
  line L86 (19.903, -0.3878) -> (18.8204, -0.3878)
  line L87 (18.8204, -0.3878) -> (18.8204, 0.2618)
  line L88 (20.5165, 0.2618) -> (21.5269, 0.2618)
  line L89 (21.5269, 0.2618) -> (21.5269, -0.3878)
  line L90 (21.5269, -0.3878) -> (20.5165, -0.3878)
  line L91 (20.5165, -0.3878) -> (20.5165, 0.2618)
  line L92 (22.0322, 0.2618) -> (23.0967, 0.2618)
  line L93 (23.0967, 0.2618) -> (23.0967, -0.3878)
  line L94 (23.0967, -0.3878) -> (22.0322, -0.3878)
  line L95 (22.0322, -0.3878) -> (22.0322, 0.2618)
  line L96 (23.6381, 0.2618) -> (24.6124, 0.2618)
  line L97 (24.6124, 0.2618) -> (24.6124, -0.3878)
  line L98 (24.6124, -0.3878) -> (23.6381, -0.3878)
  line L99 (23.6381, -0.3878) -> (23.6381, 0.2618)
  line L100 (25.13, 0.2618) -> (26.1281, 0.2618)
  line L101 (26.1281, 0.2618) -> (26.1281, -0.3878)
  line L102 (26.1281, -0.3878) -> (25.13, -0.3878)
  line L103 (25.13, -0.3878) -> (25.13, 0.2618)
  point P0 (0, 0)
  constraints: 208 end point, 63 point on line, 52 parallel, 26 horizontal, 26 perpendicular
extrude "Extrusion7" cut sketch "Sketch5" against normal blind 1 bodies 1
sketch "Sketch6" plane through (0, 1, 0) normal (0, 1, 0) x (1, 0, 0)
  line L0 (27, 13) -> (26, 13)
  line L1 (26, 13) -> (26, 12)
  line L2 (26, 12) -> (27, 12)
  line L3 (27, 12) -> (27, 13)
  line L4 (26, 12) -> (20, 12)
  line L5 (20, 12) -> (20, 4)
  line L6 (20, 4) -> (26, 4)
  line L7 (26, 4) -> (26, 12)
  line L8 (18.5, 12) -> (10.5, 12)
  line L9 (10.5, 12) -> (10.5, 4)
  line L10 (10.5, 4) -> (18.5, 4)
  line L11 (18.5, 4) -> (18.5, 12)
  point P0 (0, 0)
  dimension "d115" = 1
  dimension "d116" = 1
  dimension "d117" = 6
  dimension "d119" = 1.5
  dimension "d120" = 8
  dimension "d121" = 8
  constraints: 24 end point, 6 parallel, 3 horizontal, 3 perpendicular
  measures "d115" distance of L2.end L1.end
  measures "d116" distance of L1.end L0.end
  measures "d117" distance of L6.end L5.end
  measures "d119" distance of L4.end L8.start
  measures "d120" distance of L10.end L9.end
  measures "d121" distance of L9.end L8.end
extrude "Extrusion8" add sketch "Sketch6" along normal blind 1 contours L7 L6 L5 L4 | L11 L10 L9 L8 bodies 1
sketch "Sketch7" plane through (0, 1, 0) normal (0, 1, 0) x (1, 0, 0)
  line L0 (0.1, 12) -> (0.85, 12)
  line L1 (0.1, 11.25) -> (0.1, 12)
  line L2 (4.25, 12) -> (0.1, 12)
  line L3 (0.1, 11.75) -> (0.1, 11.34)
  line L4 (1.01, 11.34) -> (4.25, 11.34)
  line L5 (4.5, 11.59) -> (4.5, 11.75)
  line L6 (0.35, 12) -> (0.76, 12)
  line L7 (0.76, 11.09) -> (0.76, 10.91)
  line L8 (0.76, 10) -> (0.35, 10)
  line L9 (0.1, 10) -> (0.1, 12)
  line L10 (0.1, 10) -> (2.69, 10)
  line L11 (3.6, 10) -> (3.6, 10.66)
  line L12 (3.6, 10.66) -> (1.01, 10.66)
  line L13 (0.1, 10.66) -> (0.1, 10.25)
  line L14 (3.35, 10.66) -> (2.94, 10.66)
  line L15 (2.94, 9.75) -> (2.94, 9.57)
  line L16 (2.94, 8.66) -> (3.6, 8.66)
  line L17 (3.6, 8.66) -> (3.6, 10.41)
  line L18 (3.35, 8.66) -> (1.01, 8.66)
  line L19 (0.1, 8.66) -> (0.1, 9.07)
  line L20 (0.35, 9.32) -> (2.69, 9.32)
  line L21 (3.6, 9.32) -> (3.6, 8.91)
  line L22 (0.1, 9.32) -> (0.76, 9.32)
  line L23 (0.76, 8.41) -> (0.76, 8.23)
  line L24 (0.76, 7.32) -> (0.35, 7.32)
  line L25 (0.1, 7.57) -> (0.1, 9.32)
  line L26 (0.1, 7.32) -> (2.69, 7.32)
  line L27 (3.6, 7.32) -> (3.6, 7.73)
  line L28 (3.35, 7.98) -> (1.01, 7.98)
  line L29 (0.1, 7.98) -> (0.1, 7.32)
  line L30 (3.6, 7.98) -> (2.94, 7.98)
  line L31 (2.94, 7.07) -> (2.94, 6.89)
  line L32 (2.94, 5.98) -> (3.35, 5.98)
  line L33 (3.6, 6.23) -> (3.6, 7.98)
  line L34 (3.6, 5.98) -> (1.01, 5.98)
  line L35 (0.1, 5.98) -> (0.1, 6.39)
  line L36 (0.35, 6.64) -> (2.69, 6.64)
  line L37 (3.6, 6.64) -> (3.6, 5.98)
  line L38 (0.35, 6.64) -> (0.76, 6.64)
  line L39 (0.76, 5.73) -> (0.76, 5.55)
  line L40 (0.76, 4.64) -> (0.1, 4.64)
  line L41 (0.1, 4.89) -> (0.1, 6.64)
  line L42 (0.35, 4.64) -> (2.69, 4.64)
  line L43 (3.6, 4.64) -> (3.6, 5.05)
  line L44 (3.35, 5.3) -> (1.01, 5.3)
  line L45 (0.1, 5.3) -> (0.1, 4.64)
  line L46 (3.6, 5.3) -> (2.94, 5.3)
  line L47 (2.94, 4.39) -> (2.94, 4.21)
  line L48 (2.94, 3.3) -> (3.5, 3.3)
  line L49 (3.6, 3.55) -> (3.6, 5.3)
  line L50 (3.35, 3.3) -> (1.01, 3.3)
  line L51 (0.1, 3.3) -> (0.1, 3.71)
  line L52 (0.35, 3.96) -> (2.69, 3.96)
  line L53 (3.6, 3.96) -> (3.6, 3.3)
  line L54 (0.2, 3.96) -> (0.76, 3.96)
  line L55 (0.76, 3.05) -> (0.76, 2.87)
  line L56 (0.76, 1.96) -> (0.35, 1.96)
  line L57 (0.1, 2.21) -> (0.1, 3.96)
  line L58 (0.2, 1.96) -> (2.69, 1.96)
  line L59 (3.6, 1.96) -> (3.6, 2.37)
  line L60 (3.5, 2.62) -> (1.01, 2.62)
  line L61 (0.1, 2.62) -> (0.1, 2.06)
  line L62 (3.35, 2.62) -> (2.94, 2.62)
  line L63 (2.94, 1.71) -> (2.94, 1.53)
  line L64 (2.94, 0.62) -> (3.6, 0.62)
  line L65 (3.6, 0.87) -> (3.6, 2.62)
  line L66 (3.35, 0.62) -> (1.01, 0.62)
  line L67 (0.1, 0.62) -> (0.1, 1.03)
  line L68 (0.35, 1.28) -> (2.69, 1.28)
  line L69 (3.6, 1.28) -> (3.6, 0.72)
  line L70 (0.1, 0.62) -> (0.76, 0.62)
  line L71 (0.76, 0.37) -> (0.76, 0.35)
  line L72 (0.51, 0.1) -> (0.35, 0.1)
  line L73 (0.1, 0.35) -> (0.1, 0.62)
  arc A0 (0.1, 0.2) -> (0.2, 0.1) centre (0.2, 0.2) ccw
  arc A1 (0.66, 0.1) -> (0.76, 0.2) centre (0.66, 0.2) ccw
  arc A2 (0.2, 1.28) -> (0.1, 1.18) centre (0.2, 1.18) ccw
  arc A3 (0.86, 0.62) -> (0.76, 0.52) centre (0.86, 0.52) ccw
  arc A4 (3.5, 0.62) -> (3.6, 0.72) centre (3.5, 0.72) ccw
  arc A5 (2.84, 1.28) -> (2.94, 1.38) centre (2.84, 1.38) ccw
  arc A6 (3.6, 2.52) -> (3.5, 2.62) centre (3.5, 2.52) ccw
  arc A7 (2.94, 1.86) -> (2.84, 1.96) centre (2.84, 1.86) ccw
  arc A8 (0.1, 2.06) -> (0.2, 1.96) centre (0.2, 2.06) ccw
  arc A9 (0.76, 2.72) -> (0.86, 2.62) centre (0.86, 2.72) ccw
  arc A10 (0.86, 3.3) -> (0.76, 3.2) centre (0.86, 3.2) ccw
  arc A11 (0.2, 3.96) -> (0.1, 3.86) centre (0.2, 3.86) ccw
  arc A12 (2.84, 3.96) -> (2.94, 4.06) centre (2.84, 4.06) ccw
  arc A13 (3.5, 3.3) -> (3.6, 3.4) centre (3.5, 3.4) ccw
  arc A14 (0.35, 1.28) -> (0.1, 1.03) centre (0.35, 1.03) ccw
  arc A15 (0.1, 0.35) -> (0.35, 0.1) centre (0.35, 0.35) ccw
  arc A16 (0.51, 0.1) -> (0.76, 0.35) centre (0.51, 0.35) ccw
  arc A17 (2.69, 1.28) -> (2.94, 1.53) centre (2.69, 1.53) ccw
  arc A18 (3.35, 0.62) -> (3.6, 0.87) centre (3.35, 0.87) ccw
  arc A19 (1.01, 0.62) -> (0.76, 0.37) centre (1.01, 0.37) ccw
  arc A20 (2.94, 1.71) -> (2.69, 1.96) centre (2.69, 1.71) ccw
  arc A21 (3.6, 2.37) -> (3.35, 2.62) centre (3.35, 2.37) ccw
  arc A22 (0.76, 2.87) -> (1.01, 2.62) centre (1.01, 2.87) ccw
  arc A23 (1.01, 3.3) -> (0.76, 3.05) centre (1.01, 3.05) ccw
  arc A24 (0.1, 2.21) -> (0.35, 1.96) centre (0.35, 2.21) ccw
  arc A25 (0.35, 3.96) -> (0.1, 3.71) centre (0.35, 3.71) ccw
  arc A26 (3.35, 3.3) -> (3.6, 3.55) centre (3.35, 3.55) ccw
  arc A27 (2.69, 3.96) -> (2.94, 4.21) centre (2.69, 4.21) ccw
  arc A28 (2.94, 4.39) -> (2.69, 4.64) centre (2.69, 4.39) ccw
  arc A29 (3.6, 5.05) -> (3.35, 5.3) centre (3.35, 5.05) ccw
  arc A30 (0.76, 5.55) -> (1.01, 5.3) centre (1.01, 5.55) ccw
  arc A31 (0.1, 4.89) -> (0.35, 4.64) centre (0.35, 4.89) ccw
  arc A32 (0.35, 6.64) -> (0.1, 6.39) centre (0.35, 6.39) ccw
  arc A33 (1.01, 5.98) -> (0.76, 5.73) centre (1.01, 5.73) ccw
  arc A34 (0.35, 6.64) -> (0.1, 6.39) centre (0.35, 6.39) ccw
  arc A35 (2.69, 6.64) -> (2.94, 6.89) centre (2.69, 6.89) ccw
  arc A36 (3.35, 5.98) -> (3.6, 6.23) centre (3.35, 6.23) ccw
  arc A37 (2.94, 7.07) -> (2.69, 7.32) centre (2.69, 7.07) ccw
  arc A38 (3.6, 7.73) -> (3.35, 7.98) centre (3.35, 7.73) ccw
  arc A39 (3.35, 8.66) -> (3.6, 8.91) centre (3.35, 8.91) ccw
  arc A40 (2.69, 9.32) -> (2.94, 9.57) centre (2.69, 9.57) ccw
  arc A41 (1.01, 8.66) -> (0.76, 8.41) centre (1.01, 8.41) ccw
  arc A42 (0.35, 9.32) -> (0.1, 9.07) centre (0.35, 9.07) ccw
  arc A43 (0.1, 7.57) -> (0.35, 7.32) centre (0.35, 7.57) ccw
  arc A44 (0.76, 8.23) -> (1.01, 7.98) centre (1.01, 8.23) ccw
  arc A45 (3.6, 10.41) -> (3.35, 10.66) centre (3.35, 10.41) ccw
  arc A46 (2.94, 9.75) -> (2.69, 10) centre (2.69, 9.75) ccw
  arc A47 (0.76, 10.91) -> (1.01, 10.66) centre (1.01, 10.91) ccw
  arc A48 (0.1, 10.25) -> (0.35, 10) centre (0.35, 10.25) ccw
  arc A49 (0.35, 12) -> (0.1, 11.75) centre (0.35, 11.75) ccw
  arc A50 (1.01, 11.34) -> (0.76, 11.09) centre (1.01, 11.09) ccw
  arc A51 (4.25, 11.34) -> (4.5, 11.59) centre (4.25, 11.59) ccw
  arc A52 (4.5, 11.75) -> (4.25, 12) centre (4.25, 11.75) ccw
  arc A53 (0.35, 1.28) -> (0.1, 1.03) centre (0.35, 1.03) ccw
  point P0 (0, 13)
  point P1 (0.1, 1.96)
  dimension "d163" = 0.1
  dimension "d164" = 0.25
  dimension "d165" = 0.25
  constraints: 148 end point, 108 point on circle, 108 tangent, 99 point on line, 54 centre point, 51 equal radius, 36 parallel, 19 horizontal, 18 perpendicular
  measures "d163" radius of A0
  measures "d164" radius of A14
  measures "d165" radius of A37
extrude "Extrusion9" cut sketch "Sketch7" against normal blind 0.1 contours L0 L2 A52 L5 A51 L4 A50 L7 A47 L12 A45 L11 L17 A39 L16 L18 A41 L23 A44 L28 A38 L27 L33 A36 L32 L34 A33 L39 A30 L44 A29 L43 L49 A26 L48 L50 A23 L55 A22 L60 A21 L59 L65 A18 L64 L66 A19 L71 A16 L72 A15 L73 L67 A14 L68 A17 L63 A20 L58 L56 A24 L57 L51 A25 L52 A27 L47 A28 L42 L40 A31 L41 L35 A32 L36 A35 L31 A37 L26 L24 A43 L25 L19 A42 L20 A40 L15 A46 L10 L8 A48 L9 L1 A49 bodies 1
extrude "Extrusion10" add sketch "Sketch7" against normal blind 0.1 separate body contours L0 L2 A52 L5 A51 L4 A50 L7 A47 L12 A45 L11 L17 A39 L16 L18 A41 L23 A44 L28 A38 L27 L33 A36 L32 L34 A33 L39 A30 L44 A29 L43 L49 A26 L48 L50 A23 L55 A22 L60 A21 L59 L65 A18 L64 L66 A19 L71 A16 L72 A15 L73 L67 A14 L68 A17 L63 A20 L58 L56 A24 L57 L51 A25 L52 A27 L47 A28 L42 L40 A31 L41 L35 A32 L36 A35 L31 A37 L26 L24 A43 L25 L19 A42 L20 A40 L15 A46 L10 L8 A48 L9 L1 A49
body "Solid1"
body "Solid2"
body "Solid3"
body "Solid4"
